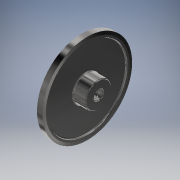
# Autodesk Inventor part: 焼結ギア
Saved by Autodesk Inventor 2019.2 (Build 232265000, 265)
## iProperties
Category: PARTsolutions
Company: KHK
Created: 2018-12-15
Part Number: 焼結ギア
Material: 鋼、高強度、低合金
Catalog Web Link: www.cadenas.de
Description: Sintered Metal Spur Gears (LS)-
Vendor: KHK
Document SubType Name: Modeling
Designer: psadmin
Manufacturer: KHK
Mass: 23.7042 g
Surface Area: 33.7151 cm^2
Volume: 3.01965 cm^3
Density: 7.85 g/cm^3
Appearance: 鋼 - つや出し
PSOL_IDENT_0: {$CADENAS_DATA\23d-libs\khk\spur_gears\sintered_metal_spur_gears_ls.prj},181 {VTYP=3D},{NB=LS0.5-80}
PSOL_IDENT_1: ,{LINA=LS0.5-80},{NN=Sintered Metal Spur Gears (LS)},{DATE=17.03.2017 04:28:21},{GEOMDATE=08.08.2007
PSOL_IDENT_2: 00:00:00},{VERSION=},{LINEID=110},{WBVAR=},{WBNUMERIC=}  {NB=LS0.5-80},{LINA=LS0.5-80},{KT=DUMMY},{
PSOL_IDENT_3: CN=LS0.5-80},{M=0.5},{Z=80},{A=4},{A1=4.1},{B=12.0},{C=40.0},{D=41.0},{E=3},{F=5},{G=8},{H=1.5},{I=0
PSOL_IDENT_4: .75},{J=36.5},{S=S9},{WMF=S9002.WMF},{L=0.2},{L2=0.23},{L3=38.35},{F1=0.00}
NN: Sintered Metal Spur Gears (LS)
NB: LS0.5-80
NBSYN: $CN.
LINA: LS0.5-80
CN: LS0.5-80
M: 0.5
Z: 80
A: 4
A1: 4.1
B: 12
C: 40
D: 41
E: 3
F: 5
G: 8
H: 1.5
I: 0.75
J: 36.5
S: S9
SUPPLIER: KHK
ARTICLENO: LS0.5-80
BOMINFO: LS0.5-80
CREATOR: CADENAS GmbH
Title: LS0.5-80
Author: Cadenas PARTsolutions
Autodesk Inventor part; units mm, degrees
ref_plane "YZ Plane" through (0, 0, 0) normal (1, 0, 0) x (0, 1, 0)
ref_plane "XZ Plane" through (0, 0, 0) normal (0, 1, 0) x (-1, 0, 0)
ref_plane "XY Plane" through (0, 0, 0) normal (0, 0, 1) x (1, 0, 0)
sketch "Sketch_2" plane through (0, 0, 0) normal (0, 0, 1) x (1, 0, 0)
  line L0 (8, 0) -> (0, 0)
  line L1 (0, 2.4) -> (0.2, 2.2)
  line L2 (0.2, 2.2) -> (0.2, 2)
  line L3 (0.2, 2) -> (6.27, 2)
  line L4 (6.27, 2) -> (6.5, 2.05)
  line L5 (6.5, 2.05) -> (7.8, 2.05)
  line L6 (7.8, 2.05) -> (7.8, 2.25)
  line L7 (7.8, 2.25) -> (8, 2.45)
  line L8 (8, 2.45) -> (8, 5.6)
  line L9 (8, 5.6) -> (7.8, 5.8)
  line L10 (7.8, 5.8) -> (7.8, 6)
  line L11 (7.8, 6) -> (3.5, 6)
  arc A0 (3, 6.5) -> (3.5, 6) centre (3.5, 6.5) ccw
  line L12 (3, 6.5) -> (3, 19.175)
  line L13 (3, 19.175) -> (2.7664, 20.5)
  line L14 (2.7664, 20.5) -> (0.2336, 20.5)
  line L15 (0.2336, 20.5) -> (0, 19.175)
  line L16 (0, 19.175) -> (0, 2.4)
  constraints: 34 end point, 2 point on circle, 1 centre point
revolve "Revolution1" add sketch "Sketch_2" angle 360 about axis through (8, 0, 0) along (1, 0, 0)
sketch "Sketch_3" plane through (0, 0, 0) normal (0, 0, 1) x (1, 0, 0)
  line L0 (0.75, 0) -> (0, 0)
  line L1 (-2, 18.25) -> (-2, 6)
  line L2 (-2, 6) -> (0, 6)
  line L3 (0, 6) -> (0.75, 6.75)
  line L4 (0.75, 6.75) -> (0.75, 17.817)
  line L5 (0.75, 17.817) -> (0, 18.25)
  line L6 (0, 18.25) -> (-2, 18.25)
  constraints: 14 end point
revolve "Revolution2" cut sketch "Sketch_3" angle 360 about axis through (0.75, 0, 0) along (1, 0, 0)
sketch "Sketch_4" plane through (0, 0, 0) normal (0, 0, 1) x (1, 0, 0)
  line L0 (3, 0) -> (2.25, 0)
  line L1 (2.25, 17.75) -> (2.25, 6.5)
  arc A0 (2.25, 6.5) -> (2.75, 6) centre (2.75, 6.5) ccw
  line L2 (2.75, 6) -> (5, 6)
  line L3 (5, 6) -> (5, 18.25)
  line L4 (5, 18.25) -> (2.75, 18.25)
  arc A1 (2.75, 18.25) -> (2.25, 17.75) centre (2.75, 17.75) ccw
  constraints: 10 end point, 4 point on circle, 2 centre point
revolve "Revolution3" cut sketch "Sketch_4" angle 360 about axis through (3, 0, 0) along (1, 0, 0)
body "Solid1"
